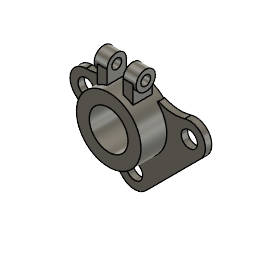
finalday26part (Autodesk Fusion 360 design; units mm, degrees)
part number: 2026-08-27-23-12-06-978
Autodesk Fusion 360 part; units mm, degrees
sketch "Sketch1" plane through (0, 0, 0) normal (0, 0, 1) x (1, 0, 0)
  circle A0 centre (0, 0) radius 30
  circle A1 centre (0, 0) radius 50
  line L0 (0, 2.5) -> (0, 20)
  circle A2 centre (84.8594, 9.9093) radius 12.5
  circle A3 centre (-74.9866, -0.0497) radius 12.5
  circle A4 centre (0.0497, -74.9866) radius 12.5
  arc A5 (27.7743, 41.5763) -> (77.8365, 33.9026) centre (61.0225, 91.3469) ccw
  arc A6 (-75.0792, 24.9502) -> (-29.9333, 40.05) centre (-75.3604, 100.8304) ccw
  line L1 (17.7522, -92.6657) -> (102.5488, -7.7567)
  line L2 (-92.6526, -17.739) -> (-17.6032, -92.6891)
  arc A7 (-17.6032, -92.6891) -> (17.7522, -92.6657) centre (0.0628, -74.9997) ccw
  arc A8 (102.5488, -7.7567) -> (77.8365, 33.9026) centre (84.8594, 9.9093) ccw
  arc A9 (-75.0792, 24.9502) -> (-92.6526, -17.739) centre (-74.9866, -0.0497) ccw
  arc A10 (-49.9951, -0.7007) -> (-49.996, 0.6345) centre (-74.9866, -0.0497) ccw
  line L3 (12.5, 0) -> (27.5, 0)
  line L4 (27.5, 0) -> (27.5, 85)
  line L5 (27.5, 85) -> (12.5, 85)
  line L6 (12.5, 85) -> (12.5, 0)
  dimension "d1" = 60
  dimension "d2" = 100
  dimension "d5" = 25
  dimension "d6" = 50
  dimension "d10" = 120
  dimension "d13" = 15
  dimension "d14" = 12.5
  dimension "d30" = 85
  constraint coincident A0.centre A1.centre
  constraint concentric A2 A8
  constraint coincident A1 A5.start
  constraint coincident A1 A6.end
  constraint tangent A1 A5
  constraint tangent A5 A8
  constraint tangent A1 A6
  constraint tangent A6 A9
  constraint tangent L1 A8
  constraint perpendicular L1 L2
  constraint tangent L2 A9
  constraint tangent L2 A7
  constraint tangent L1 A7
  constraint coincident A1 A10.end
  constraint coincident A1 A10.start
  constraint concentric A9 A10
  constraint horizontal L3
  constraint vertical L4
  constraint horizontal L5
  constraint vertical L6
  measures "d1" diameter of A0
  measures "d2" diameter of A1
  measures "d5" diameter of A2
  measures "d6" diameter of A8
  measures "d10" distance of L1.start L1.end
  measures "d13" distance of L3.start L3.end
  measures "d14" distance of A0.centre L6
  measures "d30" distance of L3.end L4.end
extrude "Extrude1" add sketch "Sketch1" along normal blind 50 contours A0 A1 A10 L4 L6 | A0 A1 L4 L6 makes body 1
extrude "Extrude2" add sketch "Sketch1" along normal blind 10 separate body contours A1 A5 A6 L1 L2 A7 A8 A9 makes body 2
fillet "Fillet1" radius 1 1 edges at (27.7743, 41.5763, 5) on bodies 2
fillet "Fillet2" radius 1 1 edges at (-29.9333, 40.05, 5) on bodies 2
extrude "Extrude3" add sketch "Sketch1" along normal blind 30 from surface at 10 separate body contours A1 L4 L5 L6 makes body 3
fillet "Fillet3" radius 15 2 edges at (20, 85, 40) (20, 85, 10) on bodies 3
cylinder "CylinderPrimitive2" add diameter 30 height 5 placed x (0, 0, -1) y (0, 1, 0) z (1, 0, 0) at (27.5, 70, 25) bodies 3
hole "Hole2" at (32.5, 70, 25) direction (-1, 0, 0) diameter 15 end through all bodies 3
mirror "Mirror1" about plane through (0, 0, 0) normal (1, 0, 0) of "Extrude3", "Fillet3", "CylinderPrimitive2", "Hole2" makes body 4
